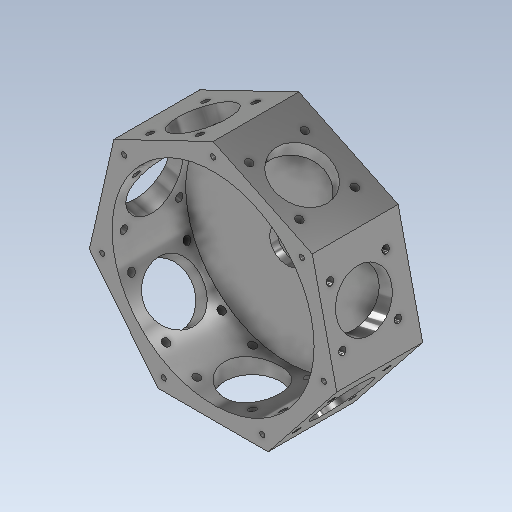
# Autodesk Inventor part: 01
Saved by Autodesk Inventor 2021 (Build 250183000, 183)
## iProperties
Category: 41
Created: 2021-07-18
Part Number: 01
Material: Liga de aço
Document SubType Name: Modeling
Designer: Giovanni
Density: 7.73 g/cm^3
Appearance: Cromado - Preto polido
User Status: 1:9
Author: Giovanni
Keywords: 1
Autodesk Inventor part; units mm, degrees
ref_plane "YZ Plane" through (0, 0, 0) normal (1, 0, 0) x (0, 1, 0)
ref_plane "XZ Plane" through (0, 0, 0) normal (0, 1, 0) x (-1, 0, 0)
ref_plane "XY Plane" through (0, 0, 0) normal (0, 0, 1) x (1, 0, 0)
sketch "Esboço1" plane through (0, 0, 0) normal (0, 0, 1) x (1, 0, 0)
  line L0 (0, 251.2194) -> (196.4112, 156.6327)
  line L1 (196.4112, 156.6327) -> (244.9208, -55.9016)
  line L2 (244.9208, -55.9016) -> (109, -226.3408)
  line L3 (109, -226.3408) -> (-109, -226.3408)
  line L4 (-109, -226.3408) -> (-244.9208, -55.9016)
  line L5 (-244.9208, -55.9016) -> (-196.4112, 156.6327)
  line L6 (-196.4112, 156.6327) -> (0, 251.2194)
  point P0 (0, 0)
  point P1 (0, 0)
  dimension "d0" = 218
  constraints: 14 end point, 1 coincident, 1 horizontal, 15 other
  measures "d0" distance of L2.end L3.end
extrude "Extrusão1" add sketch "Esboço1" along normal blind 170
sketch "Esboço2" plane through (0, 0, 170) normal (0, 0, 1) x (1, 0, 0)
  circle A0 centre (0, 0) radius 200
  dimension "d3" = 400
  constraints: 1 centre point, 1 coincident
  measures "d3" diameter of A0
extrude "Extrusão2" cut sketch "Esboço2" against normal blind 146
sketch "Esboço3" plane through (244.9208, -55.9016, 170) normal (0.7818315, -0.6234898, 0) x (0, 0, -1)
  circle A0 centre (78, -109) radius 55
  line L0 (0, -218) -> (0, 0) projected
  point P0 (170, -109)
  dimension "d6" = 110
  dimension "d7" = 78
  constraints: 1 centre point
  measures "d6" diameter of A0
  measures "d7" distance from line of L0 A0.centre
extrude "Extrusão3" cut sketch "Esboço3" against normal blind 60
sketch "Esboço4" plane through (244.9208, -55.9016, 170) normal (0.7818315, -0.6234898, 0) x (0, 0, -1)
  circle A0 centre (78, -109) radius 55 projected
  point P0 (170, -109)
  point P1 (23, -164)
  point P2 (23, -54)
  point P3 (133, -54)
  point P4 (133, -164)
  dimension "d10" = 55
  dimension "d11" = 55
  dimension "d12" = 55
  dimension "d13" = 55
  constraints: 2 horizontal alignment, 2 vertical alignment
  measures "d10" horizontal distance of A0.centre point (23, -164)
  measures "d11" horizontal distance of A0.centre point (23, -54)
  measures "d12" horizontal distance of A0.centre point (23, -54)
  measures "d13" horizontal distance of point (133, -54) A0.centre
hole "Furo1" at (142.6684, -184.1219, 147) at (211.2523, -98.1205, 147) at (211.2523, -98.1205, 37) at (142.6684, -184.1219, 37) direction (-0.7818315, 0.6234898, 0) diameter 14.376 depth 50 tip angle 118 thread size "M16x1.5" class "6H" standard "ANSI Metric M Profile"
sketch "Esboço5" plane through (-109, -226.3408, 0) normal (0, -1, 0) x (1, 0, 0)
  line L0 (109, 0) -> (109, 170) projected
  circle A0 centre (109, 92) radius 55
  line L1 (0, 170) -> (218, 170) projected
  dimension "d25" = 110
  dimension "d26" = 78
  constraints: 1 centre point, 1 point on line
  measures "d25" diameter of A0
  measures "d26" distance from line of L1 A0.centre
extrude "Extrusão4" cut sketch "Esboço5" against normal blind 60
sketch "Esboço6" plane through (-109, -226.3408, 0) normal (0, -1, 0) x (1, 0, 0)
  circle A0 centre (109, 92) radius 55 projected
  point P0 (109, 0)
  point P1 (54, 147)
  point P2 (164, 147)
  point P3 (164, 37)
  point P4 (54, 37)
  dimension "d29" = 55
  dimension "d30" = 55
  dimension "d31" = 55
  dimension "d32" = 55
  dimension "d33" = 55
  dimension "d34" = 55
  dimension "d35" = 55
  dimension "d36" = 55
  measures "d29" horizontal distance of A0.centre point (54, 147)
  measures "d30" horizontal distance of point (164, 147) A0.centre
  measures "d31" horizontal distance of A0.centre point (164, 147)
  measures "d32" horizontal distance of point (164, 37) A0.centre
  measures "d33" horizontal distance of point (164, 37) A0.centre
  measures "d34" horizontal distance of A0.centre point (54, 37)
  measures "d35" horizontal distance of A0.centre point (54, 37)
  measures "d36" horizontal distance of point (54, 147) A0.centre
hole "Furo2" at (-55, -226.3408, 147) at (55, -226.3408, 147) at (55, -226.3408, 37) at (-55, -226.3408, 37) direction (0, 1, 0) diameter 14.376 depth 50 tip angle 118 thread size "M16x1.5" class "6H" standard "ANSI Metric M Profile"
sketch "Esboço7" plane through (-109, -226.3408, 0) normal (-0.7818315, -0.6234898, 0) x (0, 0, 1)
  circle A0 centre (92, 109) radius 55
  line L0 (170, 218) -> (170, 0) projected
  point P0 (0, 109)
  dimension "d44" = 110
  dimension "d45" = 78
  constraints: 1 centre point
  measures "d44" diameter of A0
  measures "d45" distance from line of L0 A0.centre
extrude "Extrusão5" cut sketch "Esboço7" against normal blind 60
sketch "Esboço8" plane through (-109, -226.3408, 0) normal (-0.7818315, -0.6234898, 0) x (0, 0, 1)
  circle A0 centre (92, 109) radius 55 projected
  point P0 (0, 109)
  point P1 (147, 164)
  point P2 (147, 54)
  point P3 (37, 54)
  point P4 (37, 164)
  dimension "d48" = 55
  dimension "d49" = 55
  dimension "d50" = 55
  dimension "d51" = 55
  constraints: 2 horizontal alignment, 2 vertical alignment
  measures "d48" horizontal distance of A0.centre point (147, 164)
  measures "d49" horizontal distance of point (147, 54) A0.centre
  measures "d50" horizontal distance of A0.centre point (147, 54)
  measures "d51" horizontal distance of point (37, 54) A0.centre
hole "Furo3" at (-211.2523, -98.1205, 147) at (-142.6684, -184.1219, 147) at (-142.6684, -184.1219, 37) at (-211.2523, -98.1205, 37) direction (0.7818315, 0.6234898, 0) diameter 14.376 depth 50 tip angle 118 thread size "M16x1.5" class "6H" standard "ANSI Metric M Profile"
sketch "Esboço9" plane through (196.4112, 156.6327, 170) normal (0.9749279, 0.2225209, 0) x (0, 0, -1)
  circle A0 centre (78, -109) radius 55
  line L0 (0, -218) -> (0, 0) projected
  point P0 (170, -109)
  dimension "d59" = 110
  dimension "d60" = 78
  constraints: 1 centre point
  measures "d59" diameter of A0
  measures "d60" distance from line of L0 A0.centre
extrude "Extrusão6" cut sketch "Esboço9" against normal blind 60
sketch "Esboço10" plane through (196.4112, 156.6327, 170) normal (0.9749279, 0.2225209, 0) x (0, 0, -1)
  circle A0 centre (78, -109) radius 55 projected
  point P0 (170, -109)
  point P1 (23, -164)
  point P2 (23, -54)
  point P3 (133, -54)
  point P4 (133, -164)
  dimension "d63" = 55
  dimension "d64" = 55
  dimension "d65" = 55
  dimension "d66" = 55
  constraints: 2 horizontal alignment, 2 vertical alignment
  measures "d63" horizontal distance of A0.centre point (23, -164)
  measures "d64" horizontal distance of point (23, -54) A0.centre
  measures "d65" horizontal distance of point (23, -54) A0.centre
  measures "d66" horizontal distance of A0.centre point (133, -54)
hole "Furo4" at (232.9046, -3.2555, 147) at (208.4273, 103.9866, 147) at (208.4273, 103.9866, 37) at (232.9046, -3.2555, 37) direction (-0.9749279, -0.2225209, 0) diameter 14.376 depth 50 tip angle 118 thread size "M16x1.5" class "6H" standard "ANSI Metric M Profile"
sketch "Esboço11" plane through (0, 251.2194, 170) normal (0.4338837, 0.9009689, 0) x (0.9009689, -0.4338837, 0)
  circle A0 centre (109, 78) radius 55
  line L0 (218, 0) -> (0, 0) projected
  point P0 (109, 170)
  dimension "d74" = 110
  dimension "d75" = 78
  constraints: 1 centre point
  measures "d74" diameter of A0
  measures "d75" distance from line of L0 A0.centre
extrude "Extrusão7" cut sketch "Esboço11" against normal blind 60
sketch "Esboço12" plane through (0, 251.2194, 170) normal (0.4338837, 0.9009689, 0) x (0.9009689, -0.4338837, 0)
  circle A0 centre (109, 78) radius 55 projected
  point P0 (109, 170)
  point P1 (164, 23)
  point P2 (54, 23)
  point P3 (54, 133)
  point P4 (164, 133)
  dimension "d61" = 60
  dimension "d78" = 55
  dimension "d79" = 55
  dimension "d80" = 55
  dimension "d81" = 55
  constraints: 2 horizontal alignment, 2 vertical alignment
  measures "d78" horizontal distance of A0.centre point (164, 23)
  measures "d79" horizontal distance of point (54, 23) A0.centre
  measures "d80" horizontal distance of point (54, 23) A0.centre
  measures "d81" horizontal distance of point (54, 133) A0.centre
hole "Furo5" at (147.7589, 180.0624, 147) at (48.6523, 227.7896, 147) at (48.6523, 227.7896, 37) at (147.7589, 180.0624, 37) direction (-0.4338837, -0.9009689, 0) diameter 14.376 depth 50 tip angle 118 thread size "M16x1.5" class "6H" standard "ANSI Metric M Profile"
sketch "Esboço13" plane through (-196.4112, 156.6327, 170) normal (-0.4338837, 0.9009689, 0) x (0.9009689, 0.4338837, 0)
  line L0 (109, 170) -> (109, 0) projected
  circle A0 centre (109, 78) radius 55
  line L1 (218, 0) -> (0, 0) projected
  dimension "d89" = 110
  dimension "d90" = 78
  constraints: 1 centre point, 1 point on line
  measures "d89" diameter of A0
  measures "d90" distance from line of L1 A0.centre
extrude "Extrusão8" cut sketch "Esboço13" against normal blind 60
sketch "Esboço14" plane through (-196.4112, 156.6327, 170) normal (-0.4338837, 0.9009689, 0) x (0.9009689, 0.4338837, 0)
  circle A0 centre (109, 78) radius 55 projected
  point P0 (109, 170)
  point P1 (164, 23)
  point P2 (54, 23)
  point P3 (54, 133)
  point P4 (164, 133)
  dimension "d93" = 55
  dimension "d94" = 55
  dimension "d95" = 55
  dimension "d96" = 55
  constraints: 2 horizontal alignment, 2 vertical alignment
  measures "d93" horizontal distance of A0.centre point (164, 23)
  measures "d94" horizontal distance of point (54, 23) A0.centre
  measures "d95" horizontal distance of point (54, 23) A0.centre
  measures "d96" horizontal distance of A0.centre point (54, 133)
hole "Furo6" at (-48.6523, 227.7896, 147) at (-147.7589, 180.0624, 147) at (-147.7589, 180.0624, 37) at (-48.6523, 227.7896, 37) direction (0.4338837, -0.9009689, 0) diameter 14.376 depth 50 tip angle 118 thread size "M16x1.5" class "6H" standard "ANSI Metric M Profile"
sketch "Esboço15" plane through (-244.9208, -55.9016, 0) normal (-0.9749279, 0.2225209, 0) x (0, 0, 1)
  line L0 (0, 109) -> (170, 109) projected
  circle A0 centre (92, 109) radius 55
  line L1 (170, 218) -> (170, 0) projected
  dimension "d104" = 110
  dimension "d105" = 78
  constraints: 1 centre point, 1 point on line
  measures "d104" diameter of A0
  measures "d105" distance from line of L1 A0.centre
extrude "Extrusão9" cut sketch "Esboço15" against normal blind 60
sketch "Esboço16" plane through (-244.9208, -55.9016, 0) normal (-0.9749279, 0.2225209, 0) x (0, 0, 1)
  circle A0 centre (92, 109) radius 55 projected
  point P0 (0, 109)
  point P1 (147, 164)
  point P2 (147, 54)
  point P3 (37, 54)
  point P4 (37, 164)
  dimension "d108" = 55
  dimension "d109" = 55
  dimension "d110" = 55
  dimension "d111" = 55
  constraints: 2 horizontal alignment, 2 vertical alignment
  measures "d108" horizontal distance of A0.centre point (147, 164)
  measures "d109" horizontal distance of point (147, 54) A0.centre
  measures "d110" horizontal distance of A0.centre point (147, 54)
  measures "d111" horizontal distance of point (37, 54) A0.centre
hole "Furo7" at (-208.4273, 103.9866, 147) at (-232.9046, -3.2555, 147) at (-232.9046, -3.2555, 37) at (-208.4273, 103.9866, 37) direction (0.9749279, -0.2225209, 0) diameter 14.376 depth 50 tip angle 118 thread size "M16x1.5" class "6H" standard "ANSI Metric M Profile"
sketch "Esboço17" plane through (0, 0, 24) normal (0, 0, 1) x (1, 0, 0)
  circle A0 centre (0, 0) radius 34
  dimension "d119" = 68
  constraints: 1 centre point, 1 coincident
  measures "d119" diameter of A0
extrude "Extrusão10" cut sketch "Esboço17" against normal blind 15
sketch "Esboço18" plane through (0, 0, 9) normal (0, 0, 1) x (1, 0, 0)
  circle A0 centre (0, 0) radius 27.5
  dimension "d122" = 55
  constraints: 1 centre point, 1 coincident
  measures "d122" diameter of A0
extrude "Extrusão11" cut sketch "Esboço18" against normal blind 10
sketch "Esboço19" plane through (0, 0, 170) normal (0, 0, 1) x (1, 0, 0)
  point P0 (0, 0)
  point P1 (0, 225)
  dimension "d125" = 225
  constraints: 1 vertical alignment
  measures "d125" distance of point (0, 225) point (0, 0)
hole "Furo8" at (0, 225, 170) direction (0, 0, -1) diameter 10.376 depth 28 tip angle 118 thread size "M12x1.5" class "6H" standard "ANSI Metric M Profile"
sketch "Esboço20" plane through (0, 0, 0) normal (0, 0, -1) x (-1, 0, 0)
  point P0 (0, 0)
  point P1 (0, 240)
  dimension "d148" = 240
  measures "d148" distance of point (0, 0) point (0, 240)
hole "Furo9" at (0, 240, 0) direction (0, 0, 1) diameter 10.376 depth 28 tip angle 118 thread size "M12x1.5" class "6H" standard "ANSI Metric M Profile"
pattern_circular "Padrão circular1" count 7 over 360 about axis through (0, 0, 170) along (0, 0, -1) of "Furo8", "Furo9"
sketch "Esboço21" plane through (0, 0, 0) normal (0, 0, -1) x (-1, 0, 0)
  circle A0 centre (0, 0) radius 187.5
  circle A1 centre (0, 0) radius 167.5
  dimension "d143" = 375
  dimension "d144" = 335
  constraints: 2 centre point, 2 coincident
  measures "d143" diameter of A0
  measures "d144" diameter of A1
extrude "Extrusão12" cut sketch "Esboço21" against normal blind 6
